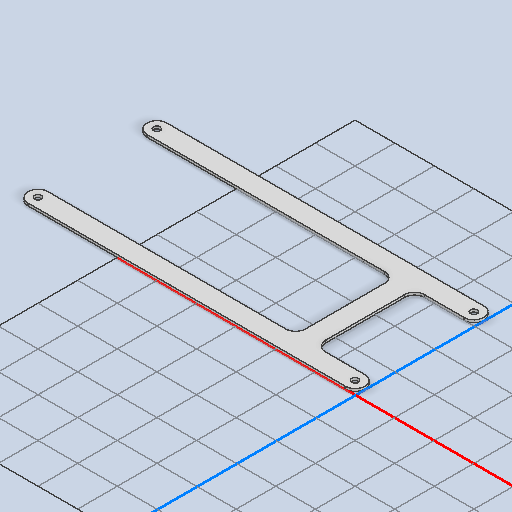
# Autodesk Inventor part: Ring Guardd
Saved by Autodesk Inventor 2026 (Build 300175000, 175)
## iProperties
Created: 2025-04-11
Part Number: Ring Guardd
Material: Generic
Document SubType Name: Modeling
Designer: avere
Density: 1 g/cm^3
Appearance: Default
Author: avere
Autodesk Inventor part; units mm, degrees
ref_plane "YZ Plane" through (0, 0, 0) normal (1, 0, 0) x (0, 1, 0)
ref_plane "XZ Plane" through (0, 0, 0) normal (0, 1, 0) x (-1, 0, 0)
ref_plane "XY Plane" through (0, 0, 0) normal (0, 0, 1) x (1, 0, 0)
sketch "Sketch1" plane through (0, 0, 0) normal (0, 1, 0) x (-1, 0, 0)
  line L0 (6.35, 0) -> (209.55, 0)
  line L1 (215.9, -6.35) -> (215.9, -6.35)
  circle A0 centre (6.35, -6.35) radius 2.1844
  circle A1 centre (209.55, -6.35) radius 2.1844
  line L2 (38.1, -19.05) -> (38.1, -69.85)
  line L3 (215.9, -82.55) -> (215.9, -82.55)
  line L4 (209.55, -88.9) -> (6.35, -88.9)
  line L5 (0, -82.55) -> (0, -82.55)
  line L6 (50.8, -19.05) -> (50.8, -69.85)
  line L7 (209.55, -12.7) -> (57.15, -12.7)
  line L8 (31.75, -12.7) -> (6.35, -12.7)
  line L9 (6.35, -76.2) -> (31.75, -76.2)
  line L10 (57.15, -76.2) -> (209.55, -76.2)
  arc A2 (57.15, -12.7) -> (50.8, -19.05) centre (57.15, -19.05) ccw
  arc A3 (38.1, -19.05) -> (31.75, -12.7) centre (31.75, -19.05) ccw
  arc A4 (31.75, -76.2) -> (38.1, -69.85) centre (31.75, -69.85) ccw
  arc A5 (50.8, -69.85) -> (57.15, -76.2) centre (57.15, -69.85) ccw
  line L11 (0, -6.35) -> (0, -6.35)
  line L12 (0, -76.2) -> (0, -88.9)
  circle A6 centre (209.55, -82.55) radius 2.1844
  circle A7 centre (6.35, -82.55) radius 2.1844
  arc A8 (215.9, -6.35) -> (209.55, 0) centre (209.55, -6.35) ccw
  arc A9 (209.55, -12.7) -> (215.9, -6.35) centre (209.55, -6.35) ccw
  arc A10 (0, -6.35) -> (6.35, -12.7) centre (6.35, -6.35) ccw
  arc A11 (6.35, 0) -> (0, -6.35) centre (6.35, -6.35) ccw
  arc A12 (6.35, -76.2) -> (0, -82.55) centre (6.35, -82.55) ccw
  arc A13 (0, -82.55) -> (6.35, -88.9) centre (6.35, -82.55) ccw
  arc A14 (215.9, -82.55) -> (209.55, -76.2) centre (209.55, -82.55) ccw
  arc A15 (209.55, -88.9) -> (215.9, -82.55) centre (209.55, -82.55) ccw
  point P0 (0, 0)
  point P1 (215.9, 0)
  point P2 (215.9, -12.7)
  point P3 (0, -12.7)
  point P4 (38.1, -12.7)
  point P5 (38.1, -76.2)
  point P6 (215.9, -76.2)
  point P7 (215.9, -88.9)
  dimension "d0" = 215.9
  dimension "d1" = 12.7
  dimension "d2" = 4.3688
  dimension "d3" = 63.5
  dimension "d4" = 12.7
  dimension "d5" = 12.7
  dimension "d6" = 38.1
  dimension "d7" = 6.35
  dimension "d8" = 6.35
  constraints: 26 end point, 24 point on circle, 24 tangent, 20 point on line, 16 centre point, 10 equal radius, 8 perpendicular, 3 horizontal, 3 vertical, 1 collinear
  measures "d0" distance of point (0, 0) point (215.9, 0)
  measures "d1" distance of point (215.9, 0) point (215.9, -12.7)
  measures "d2" diameter of A0
  measures "d3" distance of point (38.1, -12.7) point (38.1, -76.2)
  measures "d4" distance of point (215.9, -76.2) point (215.9, -88.9)
  measures "d5" distance between parallel lines of L2 L6
  measures "d6" distance from line of point (0, -12.7) L2
  measures "d7" radius of A2
  measures "d8" radius of A8
extrude "Extrusion1" add sketch "Sketch1" along normal blind 1.5875
body "Solid1"
